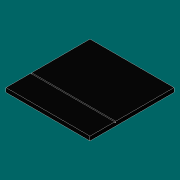
# Autodesk Inventor part: bottom
Saved by Autodesk Inventor 2016 (Build 200138000, 138)
## iProperties
Created: 2015-10-13
Part Number: bottom
Material: PC/ABS Plastic
Document SubType Name: Modeling
Designer: Sawaiz
Density: 0.357273 g/cm^3
Appearance: Smooth - Black
Author: Sawaiz
Autodesk Inventor part; units mm, degrees
ref_plane "YZ Plane" through (0, 0, 0) normal (1, 0, 0) x (0, 1, 0)
ref_plane "XZ Plane" through (0, 0, 0) normal (0, 1, 0) x (-1, 0, 0)
ref_plane "XY Plane" through (0, 0, 0) normal (0, 0, 1) x (1, 0, 0)
sketch "Sketch1" plane through (0, 0, 0) normal (0, 0, 1) x (1, 0, 0)
  line L0 (-73.025, -63.5) -> (73.025, -63.5)
  line L1 (73.025, -63.5) -> (73.025, 63.5)
  line L2 (73.025, 63.5) -> (-73.025, 63.5)
  line L3 (-73.025, 63.5) -> (-73.025, -63.5)
  line L4 (-73.025, -63.5) -> (73.025, 63.5) construction
  line L5 (73.025, -63.5) -> (-73.025, 63.5) construction
  point P0 (0, 0)
  dimension "d0" = 146.05
  dimension "d1" = 127
  constraints: 12 end point, 2 midpoint, 2 parallel, 1 horizontal, 1 perpendicular
  measures "d0" distance of L2.end L1.end
  measures "d1" distance of L1.end L0.end
extrude "Extrusion1" add sketch "Sketch1" along normal blind 6.35
sketch "Sketch13" plane through (0, 0, 6.35) normal (0, 0, 1) x (1, 0, 0)
  line L0 (-73.025, -63.5) -> (73.025, -63.5) projected
  line L1 (73.025, -63.5) -> (73.025, 63.5) projected
  line L2 (73.025, 63.5) -> (-73.025, 63.5) projected
  line L3 (-73.025, 63.5) -> (-73.025, -63.5) projected
  line L4 (-73.025, -63.5) -> (73.025, -63.5) projected
  line L5 (35.7188, -63.5) -> (34.1313, -63.5)
  line L6 (34.1313, -63.5) -> (34.1313, 63.5)
  line L7 (34.1313, 63.5) -> (35.7188, 63.5)
  line L8 (35.7188, 63.5) -> (35.7188, -63.5)
  point P0 (0, 0)
  dimension "d96" = 1.5875
  dimension "d97" = 37.3062
  constraints: 8 end point, 2 parallel, 2 point on line, 1 horizontal, 1 perpendicular
  measures "d96" distance between parallel lines of L6 L8
  measures "d97" distance between parallel lines of L1 L8
extrude "Extrusion7" cut sketch "Sketch13" against normal blind 1.5875 contours L6 L2 L8 L0
equation "\"d0\" = depth"
equation "\"d1\" = width"
equation "\"d2\" = plasticThickness"
equation "\"d97\" = aerogelHolderDepth"
equation "\"d98\" = 0.25 * plasticThickness"
equation "\"width\" = 127"
equation "\"depth\" = 146.05"
equation "\"frameAcrylicThickness\" = 9.525"
equation "\"internalAcrylicThickness\" = 6.35"
equation "\"height\" = 127"
equation "\"mirrorAngle\" = 5deg"
equation "\"detectorWidth\" = 52"
equation "\"detectorHeight\" = 52"
equation "\"mirrorThickness\" = 3.175"
equation "\"fresnelThickness\" = 0.1"
equation "\"focalLength\" = 76.2"
equation "\"ior\" = 1.49"
equation "\"centerThickness\" = 1.524"
equation "\"fresnelAngle\" = 90deg"
equation "\"fresnelEffectiveDiameter\" = 152.4"
equation "\"oRingWidth\" = 1.5875"
equation "\"sensorHolderDepth\" = 19.05"
equation "\"aerogelClearence\" = 3.175"
equation "\"backplaneHoleOffsett\" = 6.35"
equation "\"backplanePCBWidth\" = 76.2"
equation "\"backplanePCBHeight\" = 76.2"
equation "\"backplanePostionOffsett\" = 12.7"
equation "\"moduleSlotClearence\" = 0.79375"
equation "\"plasticThickness\" = 6.35"
equation "\"aerogelHolderDepth\" = 37.30625"
body "Solid1"
